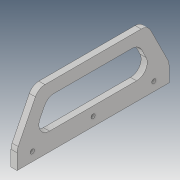
# Autodesk Inventor part: handle
Saved by Autodesk Inventor 2018 (Build 220112000, 112)
## iProperties
Created: 2020-02-09
Part Number: handle
Material: Generic
Document SubType Name: Modeling
Designer: anirudh
Density: 1 g/cm^3
Appearance: Default
Author: anirudh
Autodesk Inventor part; units mm, degrees
ref_plane "YZ Plane" through (0, 0, 0) normal (1, 0, 0) x (0, 1, 0)
ref_plane "XZ Plane" through (0, 0, 0) normal (0, 1, 0) x (-1, 0, 0)
ref_plane "XY Plane" through (0, 0, 0) normal (0, 0, 1) x (1, 0, 0)
sketch "Sketch1" plane through (0, 0, 0) normal (1, 0, 0) x (0, 1, 0)
  line L0 (0, 0) -> (0, -101.6)
  line L1 (-15, 0) -> (-15, -101.6)
  line L2 (25.4, -50.8) -> (25.4, -12.7)
  line L3 (25.4, -50.8) -> (25.4, -88.9)
  line L4 (25.4, -88.9) -> (0, -101.6)
  line L5 (25.4, -12.7) -> (0, 0)
  line L6 (-15, 0) -> (-15, 12.7)
  line L7 (-15, 12.7) -> (0, 12.7)
  line L8 (35.56, -5.08) -> (35.56, -96.52)
  line L9 (0, 12.7) -> (35.56, -5.08)
  line L10 (-15, -101.6) -> (-15, -114.3)
  line L11 (-15, -114.3) -> (0, -114.3)
  line L12 (0, -114.3) -> (35.56, -96.52)
  circle A0 centre (-7.5, 0) radius 1.75
  circle A1 centre (-7.5, -50.8) radius 1.75
  circle A2 centre (-7.5, -101.6) radius 1.75
  constraints: 26 end point, 4 vertical, 3 centre point, 2 perpendicular, 1 parallel
extrude "Extrusion1" add sketch "Sketch1" along normal blind 5.08
fillet "Fillet1" radius 8.89 8 edges at (2.54, 0, 12.7) (2.54, 35.56, -5.08) (2.54, 35.56, -96.52) (2.54, 0, -114.3) (2.54, 25.4, -12.7) (2.54, 0, 0) (2.54, 0, -101.6) (2.54, 25.4, -88.9)
body "Solid1"
